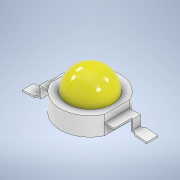
# Autodesk Inventor part: COB5730
Saved by Autodesk Inventor 2020 (Build 240168000, 168)
## iProperties
Created: 2020-03-31
Part Number: COB5730
Material: 常规
Document SubType Name: Modeling
Designer: John
Density: 1 g/cm^3
Appearance: 默认
Author: John
Autodesk Inventor part; units mm, degrees
ref_plane "YZ Plane" through (0, 0, 0) normal (1, 0, 0) x (0, 1, 0)
ref_plane "XZ Plane" through (0, 0, 0) normal (0, 1, 0) x (-1, 0, 0)
ref_plane "XY Plane" through (0, 0, 0) normal (0, 0, 1) x (1, 0, 0)
sketch "草图1" plane through (0, 0, 0) normal (0, 0, 1) x (1, 0, 0)
  line L0 (0, 0) -> (4, 0)
  line L1 (4, 0) -> (4, 2.5)
  line L2 (4, 2.5) -> (0, 2.5)
  line L3 (0, 2.5) -> (0, 0)
  line L4 (0, 2.5) -> (0, 5.5)
  arc A0 (3, 2.5) -> (0, 5.5) centre (0, 2.5) ccw
  dimension "d0" = 4
  dimension "d1" = 2.5
  dimension "d2" = 3
  constraints: 10 end point, 2 parallel, 2 point on circle, 1 centre point, 1 coincident, 1 horizontal, 1 perpendicular, 1 point on line, 1 vertical
  measures "d0" distance of L2.end L1.end
  measures "d1" distance of L1.end L0.end
  measures "d2" distance of L2.end L4.end
revolve "旋转1" add sketch "草图1" angle 360 about axis through (0, 2.5, 0) along (0, -1, 0)
sketch "草图2" plane through (0, 0, 0) normal (0, -1, 0) x (1, 0, 0)
  circle A0 centre (0, 0) radius 4 projected
  line L0 (3.63, 1.6802) -> (3.63, -1.6802)
  circle A1 centre (0, 0) radius 4 projected
  line L1 (0, 0) -> (0, -4) construction
  line L2 (-3.63, 1.6802) -> (-3.63, -1.6802)
  dimension "d4" = 3.63
  constraints: 6 end point, 2 point on circle, 2 symmetric about line, 2 vertical, 2 other
  measures "d4" distance from line of point (0, 0) L0
extrude "拉伸1" cut sketch "草图2" against normal through all contours A0 L0 | L2 A0
sketch "草图3" plane through (0, 0, 0) normal (0, -1, 0) x (1, 0, 0)
  circle A0 centre (0, 0) radius 3
  dimension "d7" = 6
  constraints: 1 centre point, 1 coincident
  measures "d7" diameter of A0
extrude "拉伸2" add sketch "草图3" along normal blind 0.2
sketch "草图4" plane through (0, 0, 0) normal (0, 0, 1) x (1, 0, 0)
  line L0 (3.63, 0) -> (3.63, 2.5) projected
  line L1 (3.63, 2.5) -> (3.63, 0) projected
  line L2 (3.63, 1.5) -> (5.1, 1.5)
  line L3 (5.1, 1.5) -> (5.1, 1.3)
  line L4 (5.1, 1.3) -> (3.63, 1.3)
  line L5 (3.63, 1.3) -> (3.63, 1.5)
  line L6 (-3.63, 2.5) -> (3.63, 2.5) projected
  line L7 (5.1, 1.5) -> (4.9, 1.5)
  line L8 (4.9, 1.5) -> (4.9, 0)
  line L9 (4.9, 0) -> (5.1, 0)
  line L10 (5.1, 0) -> (5.1, 1.5)
  line L11 (7.2, 0) -> (7.2, -0.2) construction
  line L12 (7.2, -0.2) -> (4.9, 0)
  line L13 (7.2, 0) -> (5.1, 0.1826)
  line L14 (7.2, 0) -> (7.2, -0.2)
  point P0 (0, 0)
  point P1 (4.9, 1.3)
  dimension "d10" = 1.47
  dimension "d11" = 1
  dimension "d12" = 0.2
  dimension "d13" = 0.2
  dimension "d14" = 1.5
  dimension "d15" = 0.2
  dimension "d16" = 2.1
  constraints: 24 end point, 5 parallel, 2 horizontal, 2 perpendicular, 2 point on line, 2 vertical
  measures "d10" distance of L3.end L4.end
  measures "d11" distance between parallel lines of L6 L2
  measures "d12" distance between parallel lines of L4 L2
  measures "d13" distance of L9.end L8.end
  measures "d14" distance of L8.end L7.end
  measures "d15" distance of L11.start L11.end
  measures "d16" distance between parallel lines of L10 L11
extrude "拉伸3" add sketch "草图4" along normal mid plane 3.8
sketch "草图5" plane through (3.63, 1.5, 1.9) normal (0, 1, 0) x (1, 0, 0)
  line L0 (0, 3.8) -> (0, 3.5802) projected
  line L1 (0, 0.2198) -> (0, 3.5802) projected
  line L2 (0, 0.2198) -> (0, 0) projected
  line L3 (1.47, 0) -> (0, 0) projected
  line L4 (1.47, 0) -> (1.47, 3.8) projected
  line L5 (0, 3.8) -> (1.47, 3.8) projected
  line L6 (1.47, 3.8) -> (1.47, 0) projected
  line L7 (3.57, 0) -> (1.47, 0) projected
  line L8 (3.57, 3.8) -> (3.57, 0) projected
  line L9 (1.47, 3.8) -> (3.57, 3.8) projected
  line L10 (3.57, 3.8) -> (1.97, 3.8)
  line L11 (1.97, 3.8) -> (1.97, 2.3)
  line L12 (1.97, 2.3) -> (3.57, 2.3)
  line L13 (3.57, 2.3) -> (3.57, 3.8)
  line L14 (0, 3.5802) -> (1.97, 3.5802) construction
  line L15 (3.57, 3.8) -> (3.57, 0) projected
  line L16 (1.97, 3.05) -> (3.57, 3.05) construction
  line L17 (1.97, 3.8) -> (1.7502, 3.5802)
  line L18 (1.7502, 3.5802) -> (0, 3.5802)
  line L19 (0, 2.5198) -> (1.97, 2.5198) construction
  line L20 (1.97, 2.3) -> (1.7502, 2.5198)
  line L21 (1.7502, 2.5198) -> (1.47, 2.5198)
  line L22 (1.47, 0) -> (1.47, 3.8) projected
  line L23 (1.27, 3.8) -> (1.27, 0) projected
  line L24 (1.47, 2.5198) -> (1.27, 2.5198)
  line L25 (0, 0.2198) -> (0, 0) projected
  line L26 (0, 0.2198) -> (1.27, 0.2198)
  point P0 (-3.63, 1.9)
  dimension "d19" = 1.6
  dimension "d20" = 1.5
  dimension "d21" = 45
  constraints: 26 end point, 9 point on line, 4 horizontal, 3 symmetric about line, 2 parallel, 2 perpendicular, 1 midpoint
  measures "d19" distance of L12.end L11.end
  measures "d20" distance of L11.end L10.end
  measures "d21" angle of L11 L17
extrude "拉伸4" cut sketch "草图5" against normal through all contours L5 L23 L18 L0 | L5 L4 L18 L23 | L26 L23 L3 L2 | L9 L17 L18 L4 | L23 L24 L4 L3 | L21 L20 L12 L8 L7 L4
pattern_circular "环形阵列1" count 2 over 360 about axis through (0, -10, 0) along (0, 1, 0) of "拉伸3", "拉伸4"
